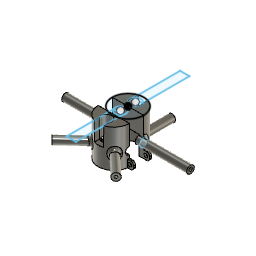
Tennis nozzle connector (Autodesk Fusion 360 design; units mm, degrees)
Autodesk Fusion 360 part; units mm, degrees
sketch "Sketch1" plane through (0, 0, 0) normal (0, 0, 1) x (1, 0, 0)
  circle A0 centre (0, 0) radius 11.65
  circle A1 centre (0, 0) radius 16.65
  dimension "d1" = 23.3
  dimension "d2" = 33.3
  constraint coincident A0.centre A1.centre
  measures "d1" diameter of A0
  measures "d2" diameter of A1
extrude "Extrude1" add sketch "Sketch1" along normal blind 20 contours A1 picked at (14.877971, -1.405965) makes body 1
ref_plane "WorkPlane1" through (0, 0, 20) normal (0, 0, 1) x (1, 0, 0)
ref_plane "WorkPlane2" through (0, 0, 40) normal (0, 0, 1) x (1, 0, 0)
sketch "Sketch4" plane through (0, 0, 40) normal (0, 0, 1) x (1, 0, 0)
  circle A0 centre (0, 0) radius 16.65
  circle A1 centre (0, 8) radius 5.65
  circle A2 centre (0, -8) radius 5.65
  line L0 (-5, -10.5) -> (5, -10.5)
  line L1 (5, -10.5) -> (5, -60.5)
  line L2 (5, -60.5) -> (-5, -60.5)
  line L3 (-5, -60.5) -> (-5, -10.5)
  line L4 (-5, 60.5) -> (5, 60.5)
  line L5 (-5, 10.5) -> (-5, 60.5)
  line L6 (5, 60.5) -> (5, 10.5)
  line L7 (5, 10.5) -> (-5, 10.5)
  dimension "d27" = 33.3
  dimension "d28" = 11.3
  dimension "d29" = 11.3
  dimension "d30" = 10
  dimension "d31" = 50
  dimension "d32" = 10
  dimension "d33" = 50
  constraint coincident A0.centre origin
  constraint horizontal L0
  constraint vertical L1
  constraint horizontal L2
  constraint vertical L3
  constraint horizontal L4
  constraint vertical L6
  constraint horizontal L7
  constraint vertical L5
  measures "d27" diameter of A0
  measures "d28" diameter of A1
  measures "d29" diameter of A2
  measures "d30" distance of L0.start L0.end
  measures "d31" distance of L0.start L2.end
  measures "d32" distance of L4.start L4.end
  measures "d33" distance of L5.start L4.start
extrude "Extrude4" add sketch "Sketch4" against normal blind 20 contours A0 A1 A2 L1 L3 L5 L6 | A0 A1 L5 L6 | A0 A2 L1 L3 | A1 L5 L6 L7 | A1 L5 L6 L7 | A2 L0 L1 L3 | A2 L0 L1 L3 picked at (-8.47312, -0.412861) picked at (-3.591124, 15.06426) picked at (-3.591124, -15.06426) picked at (0.136284, 11.545063) picked at (-0.046399, 7.783905) picked at (-0.046399, -7.783905) picked at (-0.136284, -11.545063) bodies 1
extrude "Extrude5" cut sketch "Sketch4" against normal blind 20 draft -0.5 contours A0 A1 L5 L6 | A0 L4 L5 L6 | A0 L1 L2 L3 | A0 A2 L1 L3 | A1 L5 L6 L7 | A1 L5 L6 L7 | A2 L0 L1 L3 | A2 L0 L1 L3 picked at (-3.591124, 15.06426) picked at (-0.338348, 45.87301) picked at (-0.338348, -45.87301) picked at (-3.591124, -15.06426) picked at (0.136284, 11.545063) picked at (-0.046399, 7.783905) picked at (-0.046399, -7.783905) picked at (-0.136284, -11.545063) bodies 1
sketch "Sketch3" plane through (0, 0, 0) normal (0, 1, 0) x (1, 0, 0)
  line L0 (15, -8) -> (23, -8)
  line L1 (23, -8) -> (23, 0)
  line L2 (23, 0) -> (15, 0)
  line L3 (15, 0) -> (15, -8)
  circle A0 centre (19, -4) radius 2
  circle A1 centre (-19, -4) radius 2
  line L4 (-23, -8) -> (-15, -8)
  line L5 (-15, -8) -> (-15, 0)
  line L6 (-15, 0) -> (-23, 0)
  line L7 (-23, 0) -> (-23, -8)
  dimension "d16" = 8
  dimension "d17" = 8
  dimension "d18" = 4
  dimension "d19" = 8
  dimension "d20" = 8
  dimension "d21" = 4
  constraint horizontal L0
  constraint vertical L1
  constraint horizontal L2
  constraint vertical L3
  constraint horizontal L4
  constraint vertical L5
  constraint horizontal L6
  constraint vertical L7
  measures "d16" distance of L0.start L0.end
  measures "d17" distance of L0.start L2.end
  measures "d18" diameter of A0
  measures "d19" distance of L4.end L4.start
  measures "d20" distance of L6.end L4.start
  measures "d21" diameter of A1
extrude "Extrude3" add sketch "Sketch3" along normal blind 2 and the other way blind 2 contours L0 L1 L2 L3 | L4 L5 L6 L7 picked at (19.04982, -7.331469) picked at (-18.95018, -7.331469) bodies 1
ref_plane "WorkPlane3" through (16.65, 0, 0) normal (1, 0, 0) x (0, 1, 0)
sketch "Sketch8" plane through (16.65, 0, 0) normal (1, 0, 0) x (0, 1, 0)
  circle A0 centre (0, 15) radius 4
  dimension "d56" = 8
  measures "d56" diameter of A0
split "Split1" by plane through (0, 0, 0) normal (0, 1, 0) bodies 1 makes body 2 at (-16.239991, 3.672221, 16)
ref_plane "WorkPlane6" through (12.165539, -11.367593, 30.230334) normal (0.730663, -0.68273829, 0) x (-0.68273829, -0.730663, 0)
sketch "Sketch13" plane through (12.165539, -11.367593, 30.230334) normal (0.730663, -0.68273829, 0) x (-0.68273829, -0.730663, 0)
  circle A0 centre (0, 15) radius 4
  dimension "d88" = 8
  measures "d88" diameter of A0
extrude "Extrude15" add sketch "Sketch13" along normal blind 30 and the other way blind 4 separate body contours A0 picked at (-1.709082, 16.19406) makes body 3
sketch "Sketch14" plane through (34.085429, -31.849741, 0) normal (0.730663, -0.68273829, 0) x (0.68273829, 0.730663, 0)
  circle A0 centre (0, 15.230334) radius 4
  circle A1 centre (0, 15.230334) radius 1.5
  dimension "d91" = 3
  constraint concentric A0 A1
  measures "d91" diameter of A1
extrude "Extrude16" cut sketch "Sketch14" against normal blind 15 contours A1 picked at (-0.348712, 16.234064) bodies 3
mirror "Mirror2" about plane through (0, 0, 0) normal (1, 0, 0) of bodies 3 makes body 4
move_body "Move1" bodies 1 4 3 to x (1, 0, 0) y (0, 1, 0) z (0, 0, 1) at (0, -15, 0)
extrude "Extrude10" add sketch "Sketch8" along normal blind 50 and the other way blind 5 separate body contours A0 picked at (0.237931, 16.042442) makes body 5
sketch "Sketch10" plane through (66.65, 0, 0) normal (1, 0, 0) x (0, 1, 0)
  circle A0 centre (0, 15) radius 4
  circle A1 centre (0, 15) radius 1.8
  dimension "d68" = 3.6
  constraint concentric A0 A1
  measures "d68" diameter of A1
extrude "Extrude12" cut sketch "Sketch10" against normal blind 20 contours A1 picked at (-0.133513, 15.454274) bodies 5
mirror "Mirror1" about plane through (0, 0, 0) normal (1, 0, 0) of bodies 5 makes body 6
sketch "Sketch9" plane through (16.65, 0, 0) normal (1, 0, 0) x (0, 1, 0)
  circle A0 centre (-15, 15) radius 4
  dimension "d65" = 8
  measures "d65" diameter of A0
extrude "Extrude11" cut sketch "Sketch9" against normal blind 33.3 contours A0 picked at (-14.565015, 16.012741) bodies 1
ref_plane "WorkPlane4" through (0, 16.65, 0) normal (0, 1, 0) x (0, 0, 1)
sketch "Sketch11" plane through (0, 16.65, 0) normal (0, 1, 0) x (1, 0, 0)
  circle A0 centre (0, -6) radius 4
  dimension "d72" = 8
  measures "d72" diameter of A0
extrude "Extrude13" add sketch "Sketch11" along normal blind 30 and the other way blind 4 separate body contours A0 picked at (-0.904125, -6.856937) makes body 7
sketch "Sketch12" plane through (0, 46.65, 0) normal (0, 1, 0) x (-1, 0, 0)
  circle A0 centre (0, 6) radius 4
  circle A1 centre (0, 6) radius 1.8
  dimension "d77" = 3.6
  constraint concentric A0 A1
  measures "d77" diameter of A1
extrude "Extrude14" cut sketch "Sketch12" against normal blind 20 contours A1 picked at (0.3, 6.519615) bodies 7
fillet "Fillet1" radius 3 8 edges at (23, -16, 8) (23, -16, 0) (-23, -16, 8) (-23, -16, 0) (23, 1, 8) (23, 1, 0) (-23, 1, 8) (-23, 1, 0) on bodies 1 2
combine "Combine2" operation add target body 2 tool bodies 7 6 5
combine "Combine3" operation add target body 1 tool bodies 4 3
fillet "Fillet3" radius 3 2 edges at (-9.078299, -28.957327, 15.230334) (9.078299, -28.957327, 15.230334) on bodies 1 2
fillet "Fillet3" radius 3 1 edges at (16.162379, 4, 15) on bodies 1 2
fillet "Fillet3" radius 2 1 edges at (4, 16.162379, 6) on bodies 1 2
fillet "Fillet3" radius 3 1 edges at (-16.162379, 4, 15) on bodies 1 2
